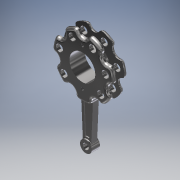
# Autodesk Inventor part: Component 2 (Connecting Rod Hub)
Saved by Autodesk Inventor 2018 (Build 220112000, 112)
## iProperties
Created: 2023-03-12
Part Number: Component 2 (Connecting Rod Hub)
Material: Generic
Document SubType Name: Modeling
Designer: Habib Mohamed
Density: 1 g/cm^3
Appearance: Silicon Nitride - Polished
Author: Habib Mohamed
Autodesk Inventor part; units mm, degrees
ref_plane "YZ Plane" through (0, 0, 0) normal (1, 0, 0) x (0, 1, 0)
ref_plane "XZ Plane" through (0, 0, 0) normal (0, 1, 0) x (-1, 0, 0)
ref_plane "XY Plane" through (0, 0, 0) normal (0, 0, 1) x (1, 0, 0)
sketch "Sketch1" plane through (0, 0, 0) normal (0, 0, 1) x (1, 0, 0)
  circle A0 centre (0, 0) radius 11
  circle A1 centre (0, 0) radius 20.98 construction
  arc A2 (-4.349128, 23.513203) -> (4.349128, 23.513203) centre (0, 25.98) ccw
  arc A3 (-4.349128, 23.513203) -> (-7.833334, 24.791912) centre (-6.845527, 22.097262) ccw
  line L0 (0, 0) -> (0, 71.630035) construction
  arc A4 (7.833334, 24.791912) -> (4.349128, 23.513203) centre (6.845527, 22.097262) ccw
  arc A5 (-21.094999, 11.259957) -> (-24.267101, 9.333157) centre (-21.544451, 8.425369) ccw
  arc A6 (-21.094999, 11.259957) -> (-15.671726, 18.060527) centre (-20.311982, 16.198265) ccw
  arc A7 (-14.499093, 21.581851) -> (-15.671726, 18.060527) centre (-13.008218, 19.129466) ccw
  arc A8 (-21.955906, -9.472266) -> (-22.427246, -13.153655) centre (-20.019964, -11.590999) ccw
  arc A9 (-21.955906, -9.472266) -> (-23.89145, -0.992094) centre (-25.328627, -5.781094) ccw
  arc A10 (-25.913407, 2.120217) -> (-23.89145, -0.992094) centre (-23.06651, 1.756792) ccw
  arc A11 (-6.283568, -23.07168) -> (-3.699217, -25.735497) centre (-3.420036, -22.879108) ccw
  arc A12 (-6.283568, -23.07168) -> (-14.120425, -19.297648) centre (-11.2723, -23.407171) ccw
  arc A13 (-17.814397, -18.937984) -> (-14.120425, -19.297648) centre (-15.755249, -16.938782) ccw
  arc A14 (14.120425, -19.297648) -> (17.814397, -18.937984) centre (15.755249, -16.938782) ccw
  arc A15 (14.120425, -19.297648) -> (6.283568, -23.07168) centre (11.2723, -23.407171) ccw
  arc A16 (3.699217, -25.735497) -> (6.283568, -23.07168) centre (3.420036, -22.879108) ccw
  arc A17 (23.89145, -0.992094) -> (25.913407, 2.120217) centre (23.06651, 1.756792) ccw
  arc A18 (23.89145, -0.992094) -> (21.955906, -9.472266) centre (25.328627, -5.781094) ccw
  arc A19 (22.427246, -13.153655) -> (21.955906, -9.472266) centre (20.019964, -11.590999) ccw
  arc A20 (15.671726, 18.060527) -> (14.499093, 21.581851) centre (13.008218, 19.129466) ccw
  arc A21 (15.671726, 18.060527) -> (21.094999, 11.259957) centre (20.311982, 16.198265) ccw
  arc A22 (24.267101, 9.333157) -> (21.094999, 11.259957) centre (21.544451, 8.425369) ccw
  arc A23 (-7.833334, 24.791912) -> (-14.499093, 21.581851) centre (0, 0) ccw
  arc A24 (-24.267101, 9.333157) -> (-25.913407, 2.120217) centre (0, 0) ccw
  arc A25 (-22.427246, -13.153655) -> (-17.814397, -18.937984) centre (0, 0) ccw
  arc A26 (-3.699217, -25.735497) -> (3.699217, -25.735497) centre (0, 0) ccw
  arc A27 (17.814397, -18.937984) -> (22.427246, -13.153655) centre (0, 0) ccw
  arc A28 (25.913407, 2.120217) -> (24.267101, 9.333157) centre (0, 0) ccw
  arc A29 (14.499093, 21.581851) -> (7.833334, 24.791912) centre (0, 0) ccw
  circle A30 centre (15.63663, -12.469796) radius 3
  line L1 (0, 0) -> (45.686533, 0) construction
  line L2 (0, 0) -> (15.63663, -12.469796) construction
  line L3 (15.63663, -12.469796) -> (20.327619, -16.210735) construction
  circle A31 centre (19.498558, 4.450419) radius 3
  circle A32 centre (8.677675, 18.019377) radius 3
  circle A33 centre (-8.677675, 18.019377) radius 3
  circle A34 centre (-19.498558, 4.450419) radius 3
  circle A35 centre (-15.63663, -12.469796) radius 3
  dimension "d0" = 22
  dimension "d2" = 41.96
  dimension "d3" = 10
  dimension "d4" = 5.74
  dimension "d7" = 360
  dimension "d9" = 26
  dimension "d10" = 6
  dimension "d11" = 20
  constraints: 57 point on circle, 36 centre point, 8 end point, 4 coincident, 2 tangent, 1 collinear, 1 horizontal, 1 symmetric about line, 1 vertical, 1 vertical alignment, 72 other
  measures "d0" diameter of A0
  measures "d2" diameter of A1
  measures "d3" diameter of A2
  measures "d4" diameter of A3
  measures "d9" radius of A23
  measures "d10" diameter of A30
  measures "d11" distance of L0.start L2.end
extrude "Extrusion1" add sketch "Sketch1" along normal blind 13
sketch "Sketch2" plane through (0, 0, 0) normal (0, 0, 1) x (1, 0, 0)
  arc A0 (6.962417, -12.145977) -> (-6.962417, -12.145977) centre (0, 0) ccw construction
  arc A1 (14.904619, -30.558998) -> (-14.904619, -30.558998) centre (0, 0) ccw construction
  line L0 (-6.560939, -13.451918) -> (-14.904619, -30.558998) construction
  line L1 (0, 0) -> (0, -45.573733) construction
  line L2 (6.560939, -13.451918) -> (14.904619, -30.558998) construction
  arc A2 (6.962417, -12.145977) -> (6.560939, -13.451918) centre (7.459733, -13.013546) ccw construction
  arc A3 (-6.560939, -13.451918) -> (-6.962417, -12.145977) centre (-7.459733, -13.013546) ccw construction
  point P0 (-15.004581, -30.763951)
  point P1 (15.004581, -30.763951)
  dimension "d17" = 28
  dimension "d18" = 26
  dimension "d19" = 34
  dimension "d20" = 26
  dimension "d23" = 2
  constraints: 8 point on circle, 6 end point, 4 centre point, 2 coincident, 2 symmetric about line, 2 tangent, 1 vertical, 1 other
  measures "d17" diameter of A0
  measures "d18" angle of L0 L1
  measures "d19" radius of A1
  measures "d20" angle of L1 L2
  measures "d23" diameter of A2
ref_plane "Work Plane1" through (0, 0, 6.5) normal (0, 0, -1) x (-1, 0, 0)
sketch "Sketch3" plane through (0, 0, 6.5) normal (0, 0, -1) x (-1, 0, 0)
  arc A0 (14.904619, -30.558998) -> (-14.904619, -30.558998) centre (0, 0) ccw
  arc A1 (-6.962417, -12.145977) -> (-6.962417, -12.145977) centre (0, 0) ccw
  line L0 (-6.560939, -13.451918) -> (-14.904619, -30.558998)
  line L1 (6.560939, -13.451918) -> (14.904619, -30.558998)
  arc A2 (-6.560939, -13.451918) -> (-6.962417, -12.145977) centre (-7.459733, -13.013546) ccw
  arc A3 (6.962417, -12.145977) -> (6.560939, -13.451918) centre (7.459733, -13.013546) ccw
  arc A4 (6.962417, -12.145977) -> (-6.962417, -12.145977) centre (0, 0) ccw
  constraints: 4 point on circle, 1 centre point, 1 coincident, 2 other
extrude "Extrusion2" cut sketch "Sketch3" along normal mid plane 7 contours L1 A3 A1 A2 L0 A0
sketch "Sketch4" plane through (0, 0, 0) normal (0, 0, 1) x (1, 0, 0)
  line L0 (0, 0) -> (0, -60) construction
  circle A0 centre (0, -60) radius 2.5 construction
  circle A1 centre (0, -60) radius 5 construction
  line L1 (-4.98, -26) -> (4.98, -26) construction
  arc A2 (-3.699217, -25.735497) -> (3.699217, -25.735497) centre (0, 0) ccw construction
  line L2 (-3.615, -55) -> (3.615, -55) construction
  line L3 (4.98, -26) -> (4.98, -25.288135) construction
  line L4 (-4.98, -26) -> (-4.98, -25.288135) construction
  line L5 (-3.615, -55) -> (-3.615, -56.54576) construction
  line L6 (3.615, -55) -> (3.615, -56.54576) construction
  line L7 (-4.98, -25.288135) -> (-3.615, -56.54576) construction
  line L8 (4.98, -25.288135) -> (3.615, -56.54576) construction
  arc A3 (3.699217, -25.735497) -> (6.283568, -23.07168) centre (3.420036, -22.879108) ccw construction
  arc A4 (-6.283568, -23.07168) -> (-3.699217, -25.735497) centre (-3.420036, -22.879108) ccw construction
  arc A5 (-2.405943, -27.826181) -> (2.405943, -27.826181) centre (0, 0) ccw construction
  arc A6 (-3.699217, -25.735497) -> (3.699217, -25.735497) centre (0, 0) ccw construction
  line L9 (2.915982, -28.314939) -> (1.829942, -53.184553) construction
  line L10 (-1.829942, -53.184553) -> (-2.915982, -28.314939) construction
  line L11 (-4.98, -27.93) -> (-4.864631, -27.93) construction
  arc A7 (1.268656, -53.625009) -> (-1.268656, -53.625009) centre (0, -60) ccw construction
  arc A8 (-3.697604, -54.654186) -> (3.697604, -54.654186) centre (0, -60) ccw construction
  arc A9 (-2.405943, -27.826181) -> (-2.915982, -28.314939) centre (-2.44643, -28.294434) ccw construction
  arc A10 (2.915982, -28.314939) -> (2.405943, -27.826181) centre (2.44643, -28.294434) ccw construction
  arc A11 (-1.829942, -53.184553) -> (-1.268656, -53.625009) centre (-1.36039, -53.164048) ccw construction
  arc A12 (1.268656, -53.625009) -> (1.829942, -53.184553) centre (1.36039, -53.164048) ccw construction
  point P0 (0, -26)
  point P1 (0, -55)
  point P2 (0, -26)
  dimension "d28" = 60
  dimension "d29" = 5
  dimension "d30" = 10
  dimension "d31" = 9.96
  dimension "d32" = 7.23
  dimension "d36" = 1.93
  dimension "d37" = 0.94
  dimension "d38" = 0.94
  dimension "d39" = 0.94
  constraints: 24 end point, 23 point on circle, 10 centre point, 8 tangent, 5 point on line, 3 midpoint, 3 parallel, 2 coincident, 2 horizontal, 2 vertical, 1 equal radius
  measures "d28" distance of L0.start L0.end
  measures "d29" diameter of A0
  measures "d30" diameter of A1
  measures "d31" distance of L1.start L1.end
  measures "d32" distance of L2.start L2.end
  measures "d36" radial gap between concentric circles of A2 A5
  measures "d37" diameter of A9
  measures "d38" diameter of A11
  measures "d39" diameter of A12
sketch "Sketch5" plane through (0, 0, 6.5) normal (0, 0, -1) x (-1, 0, 0)
  circle A0 centre (0, -60) radius 5
  circle A1 centre (0, -60) radius 2.5
  line L0 (-4.98, -25.288135) -> (-3.615, -56.54576)
  line L1 (4.98, -25.288135) -> (3.615, -56.54576)
  line L2 (1.829942, -53.184553) -> (2.915982, -28.314939)
  line L3 (-2.915982, -28.314939) -> (-1.829942, -53.184553)
  arc A2 (1.268656, -53.625009) -> (-1.268656, -53.625009) centre (0, -60) ccw
  arc A3 (1.268656, -53.625009) -> (1.829942, -53.184553) centre (1.36039, -53.164048) ccw
  arc A4 (-1.829942, -53.184553) -> (-1.268656, -53.625009) centre (-1.36039, -53.164048) ccw
  arc A5 (2.915982, -28.314939) -> (2.405943, -27.826181) centre (2.44643, -28.294434) ccw
  arc A6 (-2.405943, -27.826181) -> (2.405943, -27.826181) centre (0, 0) ccw
  arc A7 (-2.405943, -27.826181) -> (-2.915982, -28.314939) centre (-2.44643, -28.294434) ccw
  arc A8 (-3.699217, -25.735497) -> (3.699217, -25.735497) centre (0, 0) ccw
  arc A9 (-6.283568, -23.07168) -> (-3.699217, -25.735497) centre (-3.420036, -22.879108) ccw
  arc A10 (3.699217, -25.735497) -> (6.283568, -23.07168) centre (3.420036, -22.879108) ccw
extrude "Extrusion3" add sketch "Sketch5" along normal mid plane 7 contours A0
extrude "Extrusion4" add sketch "Sketch5" along normal mid plane 5 contours A0 L0 A9 A8 A10 L1 | A3 A2 A4 L3 A7 A6 A5 L2
sketch "Sketch6" plane through (0, 0, 10) normal (0, 0, 1) x (1, 0, 0)
  arc A0 (-2.405943, -27.826181) -> (2.405943, -27.826181) centre (0, 0) ccw construction
  arc A1 (2.915982, -28.314939) -> (2.405943, -27.826181) centre (2.44643, -28.294434) ccw construction
  line L0 (2.915982, -28.314939) -> (1.829942, -53.184553) construction
  arc A2 (-2.405943, -27.826181) -> (-2.915982, -28.314939) centre (-2.44643, -28.294434) ccw construction
  line L1 (-1.829942, -53.184553) -> (-2.915982, -28.314939) construction
  arc A3 (1.268656, -53.625009) -> (1.829942, -53.184553) centre (1.36039, -53.164048) ccw construction
  arc A4 (1.268656, -53.625009) -> (-1.268656, -53.625009) centre (0, -60) ccw construction
  arc A5 (-1.829942, -53.184553) -> (-1.268656, -53.625009) centre (-1.36039, -53.164048) ccw construction
sketch "Sketch7" plane through (0, 0, 13) normal (0, 0, 1) x (1, 0, 0)
  point P0 (0, 0)
  point P1 (0, 16)
  point P2 (0, -16)
  dimension "d46" = 16
  dimension "d47" = 16
  measures "d46" distance of point (0, 0) point (0, 16)
  measures "d47" distance of point (0, -16) point (0, 0)
hole "Hole1" at (0, 16, 13) at (0, -16, 13) direction (0, 0, -1) diameter 2.459 depth 16.55 tip angle 118 thread size "M3x0.5" class "6H" standard "ISO Metric profile"
fillet "Fillet1" radius 2.5 56 edges at (5.8567, 24.7915, 13) (0, 20.98, 13) (-5.8567, 24.7915, 13) (-11.281, 23.4252, 13) (-15.7312, 20.0362, 13) (-16.4028, 13.0808, 13) (-23.0344, 10.8783, 13) (-25.3481, 5.7855, 13) (-25.4732, 0.1932, 13) (-20.454, -4.6685, 13) (-22.8667, -11.2265, 13) (-20.3276, -16.2107, 13) (-16.0334, -19.7953, 13) (-9.1029, -18.9023, 13) (-5.4799, -24.8775, 13) (0, -26, 13) (5.4799, -24.8775, 13) (9.1029, -18.9023, 13) (16.0334, -19.7953, 13) (20.3276, -16.2107, 13) (22.8667, -11.2265, 13) (20.454, -4.6685, 13) (25.4732, 0.1932, 13) (25.3481, 5.7855, 13) (23.0344, 10.8783, 13) (16.4028, 13.0808, 13) (15.7312, 20.0362, 13) (11.281, 23.4252, 13) (5.8567, 24.7915, 0) (11.281, 23.4252, 0) (15.7312, 20.0362, 0) (16.4028, 13.0808, 0) (23.0344, 10.8783, 0) (25.3481, 5.7855, 0) (25.4732, 0.1932, 0) (20.454, -4.6685, 0) (22.8667, -11.2265, 0) (20.3276, -16.2107, 0) (16.0334, -19.7953, 0) (9.1029, -18.9023, 0) (5.4799, -24.8775, 0) (0, -26, 0) (-5.4799, -24.8775, 0) (-9.1029, -18.9023, 0) (-16.0334, -19.7953, 0) (-20.3276, -16.2107, 0) (-22.8667, -11.2265, 0) (-20.454, -4.6685, 0) (-25.4732, 0.1932, 0) (-25.3481, 5.7855, 0) (-23.0344, 10.8783, 0) (-16.4028, 13.0808, 0) (-15.7312, 20.0362, 0) (-11.281, 23.4252, 0) (-5.8567, 24.7915, 0) (0, 20.98, 0)
sketch "Sketch8" plane through (0, 0, 9) normal (0, 0, 1) x (1, 0, 0)
  line L0 (-1.829942, -53.184553) -> (-2.915982, -28.314939)
  arc A0 (-2.405943, -27.826181) -> (2.405943, -27.826181) centre (0, 0) ccw
  arc A1 (-2.405943, -27.826181) -> (-2.915982, -28.314939) centre (-2.44643, -28.294434) ccw
  line L1 (2.915982, -28.314939) -> (1.829942, -53.184553)
  arc A2 (2.915982, -28.314939) -> (2.405943, -27.826181) centre (2.44643, -28.294434) ccw
  arc A3 (-1.829942, -53.184553) -> (-1.268656, -53.625009) centre (-1.36039, -53.164048) ccw
  arc A4 (1.268656, -53.625009) -> (-1.268656, -53.625009) centre (0, -60) ccw
  arc A5 (1.268656, -53.625009) -> (1.829942, -53.184553) centre (1.36039, -53.164048) ccw
extrude "Extrusion6" cut sketch "Sketch8" against normal blind 0.88
mirror "Mirror2" about plane through (0, 0, 6.5) normal (0, 0, -1) of "Extrusion6"
fillet "Fillet2" radius 0.5 4 edges at (3.615, -56.5458, 6.5) (0, -55, 9) (0, -55, 4) (-3.615, -56.5458, 6.5)
fillet "Fillet3" radius 0.85 8 edges at (4.3664, -25.5886, 9) (0, -26, 9) (-4.3664, -25.5886, 9) (4.98, -25.2881, 6.5) (4.3664, -25.5886, 4) (0, -26, 4) (-4.3664, -25.5886, 4) (-4.98, -25.2881, 6.5)
equation "\"d47\" = d46"
body "Solid1"
